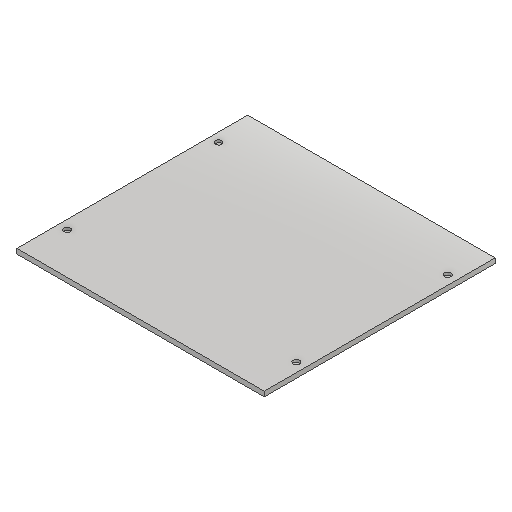
# Autodesk Inventor part: CNCM_ALU_6mm_Heatbed
Saved by Autodesk Inventor 2026.1 (Build 301233000, 233)
## iProperties
Created: 2017-05-24
Part Number: CNCM_ALU_6mm_Heatbed
Material: Ogólny
Document SubType Name: Modeling
Designer: Andrzej
Density: 1 g/cm^3
Appearance: Aluminium — polerowane
Author: Andrzej
Autodesk Inventor part; units mm, degrees
ref_plane "YZ Plane" through (0, 0, 0) normal (1, 0, 0) x (0, 1, 0)
ref_plane "XZ Plane" through (0, 0, 0) normal (0, 1, 0) x (-1, 0, 0)
ref_plane "XY Plane" through (0, 0, 0) normal (0, 0, 1) x (1, 0, 0)
sketch "Szkic1" plane through (0, 0, 0) normal (0, 0, 1) x (1, 0, 0)
  line L0 (-13.9027, 6.9311) -> (286.0973, 6.9311)
  line L1 (286.0973, 6.9311) -> (286.0973, -273.0689)
  line L2 (286.0973, -273.0689) -> (-13.9027, -273.0689)
  line L3 (-13.9027, -273.0689) -> (-13.9027, 6.9311)
  point P0 (0, 0)
  dimension "d0" = 300
  dimension "d1" = 280
  constraints: 8 end point, 2 parallel, 1 horizontal, 1 perpendicular
  measures "d0" distance of L1.end L2.end
  measures "d1" distance of L0.end L1.end
extrude "Wyciągnięcie proste1" add sketch "Szkic1" along normal blind 6
sketch "Szkic2" plane through (0, 0, 6) normal (0, 0, 1) x (1, 0, 0)
  line L0 (286.0973, 6.9311) -> (-13.9027, 6.9311) projected
  line L1 (-13.9027, 6.9311) -> (-13.9027, -273.0689) projected
  line L2 (-13.9027, -273.0689) -> (286.0973, -273.0689) projected
  line L3 (286.0973, -273.0689) -> (286.0973, 6.9311) projected
  point P0 (0, 0)
  point P1 (-2.9027, -39.5689)
  point P2 (275.0973, -39.5689)
  point P3 (-2.9027, -223.0689)
  point P4 (275.0973, -223.0689)
  dimension "d4" = 46.5
  dimension "d5" = 300
  dimension "d6" = 46.5
  dimension "d7" = 11
  dimension "d8" = 11
  dimension "d9" = 50
  dimension "d10" = 50
  dimension "d11" = 11
  dimension "d12" = 11
  measures "d4" distance from line of L0 point (-2.903, -39.569)
  measures "d5" distance between parallel lines of L3 L1
  measures "d6" distance from line of L0 point (275.097, -39.569)
  measures "d7" distance from line of L3 point (275.097, -39.569)
  measures "d8" distance from line of L1 point (-2.903, -39.569)
  measures "d9" distance from line of L2 point (-2.903, -223.069)
  measures "d10" distance from line of L2 point (275.097, -223.069)
  measures "d11" distance from line of L1 point (-2.903, -223.069)
  measures "d12" distance from line of L3 point (275.097, -223.069)
hole "Otwór1" at (-2.9027, -39.5689, 6) at (275.0973, -39.5689, 6) at (-2.9027, -223.0689, 6) at (275.0973, -223.0689, 6) direction (0, 0, -1) diameter 4 end through all
hole "Otwór2" at (-2.9027, -39.5689, 6) at (275.0973, -39.5689, 6) at (-2.9027, -223.0689, 6) at (275.0973, -223.0689, 6) direction (0, 0, -1) diameter 8 depth 3 tip angle 118
equation "\"d6\" = d4"
equation "\"d7\" = d8"
equation "\"d11\" = d8"
equation "\"d12\" = d8"
